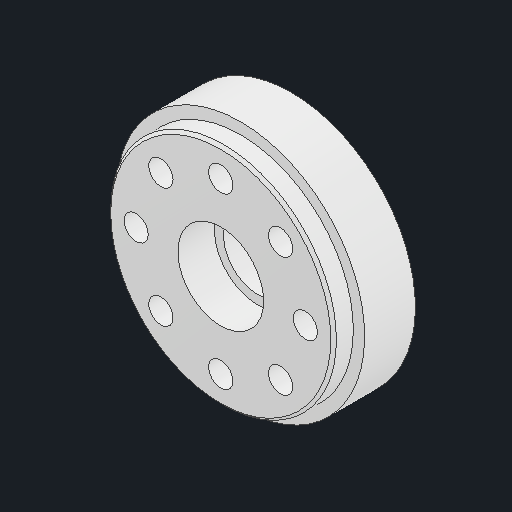
# Autodesk Inventor part: scara-base16
Saved by Autodesk Inventor 2022 (Build 260153000, 153)
## iProperties
Created: 2021-10-10
Part Number: scara-base16
Material: ABS プラスチック
Document SubType Name: Modeling
Designer: Yuta Kage
Density: 1.06 g/cm^3
Appearance: 滑らか - 白
Mass: 19.5117 g
Surface Area: 70.0236 cm^2
Volume: 18.4073 cm^3
Description: 印刷
Author: Yuta Kage
Autodesk Inventor part; units mm, degrees
ref_plane "YZ Plane" through (0, 0, 0) normal (1, 0, 0) x (0, 1, 0)
ref_plane "XZ Plane" through (0, 0, 0) normal (0, 1, 0) x (-1, 0, 0)
ref_plane "XY Plane" through (0, 0, 0) normal (0, 0, 1) x (1, 0, 0)
sketch "スケッチ1" plane through (0, 0, 0) normal (1, 0, 0) x (0, 1, 0)
  line L0 (0, 0) -> (20, 0)
  line L1 (20, 0) -> (20, -3.5)
  line L2 (20, -3.5) -> (22, -3.5)
  line L3 (22, -3.5) -> (22, -12.5)
  line L4 (22, -12.5) -> (0, -12.5)
  line L5 (0, -12.5) -> (0, 0)
  line L6 (12, 0) -> (12, -12.5)
  dimension "d0" = 20
  dimension "d1" = 2
  dimension "d23" = 12
  dimension "d35" = 3.5
  dimension "d40" = 9
  constraints: 14 end point, 6 perpendicular, 2 point on line, 1 horizontal
  measures "d0" distance of L0.start L0.end
  measures "d1" distance of L1.end L2.end
  measures "d23" distance between parallel lines of L5 L6
  measures "d35" distance of L0.end L1.end
  measures "d40" distance of L2.end L3.end
revolve "回転1" add sketch "スケッチ1" angle 360 about axis through (0, 0, -12.5) along (0, 0, 1)
chamfer "面取り1" distance 0.5 angle 45 1 edges at (0, -20, 0)
sketch "スケッチ4" plane through (0, 0, -12.5) normal (0, 0, -1) x (-1, 0, 0)
  circle A0 centre (0, 0) radius 15
  point P0 (0, 15)
  point P1 (-10.6066, 10.6066)
  point P2 (-15, 0)
  point P3 (-10.6066, -10.6066)
  point P4 (0, -15)
  point P5 (10.6066, -10.6066)
  point P6 (15, 0)
  point P7 (10.6066, 10.6066)
  dimension "d41" = 30
  dimension "d44" = 360
  constraints: 1 vertical alignment, 11 other
hole "穴2" at (-10.6066, 10.6066, -12.5) at (-15, 0, -12.5) at (-10.6066, -10.6066, -12.5) at (0, -15, -12.5) at (10.6066, -10.6066, -12.5) at (15, 0, -12.5) at (10.6066, 10.6066, -12.5) at (0, 15, -12.5) direction (0, 0, 1) diameter 4.3 end through all counterbore diameter 8 counterbore depth 2 clearance for "Socket Head Cap Screw" size "M4" standard "Ansi Metric M Profile"
sketch "スケッチ6" plane through (0, 0, 0) normal (0, 0, 1) x (1, 0, 0)
  circle A0 centre (0, 0) radius 7.6
  point P0 (0, 0)
  dimension "d46" = 15.2
  constraints: 1 centre point, 1 coincident
  measures "d46" diameter of A0
extrude "押し出し3" cut sketch "スケッチ6" against normal blind 6.5
sketch "スケッチ7" plane through (0, 0, -6.5) normal (0, 0, 1) x (1, 0, 0)
  circle A0 centre (0, 0) radius 6
  point P0 (0, 0)
  dimension "d49" = 12
  constraints: 1 centre point, 1 coincident
  measures "d49" diameter of A0
extrude "押し出し4" cut sketch "スケッチ7" against normal through all
